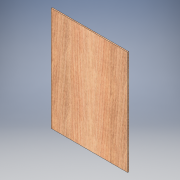
# Autodesk Inventor part: testBasePlate
Saved by Autodesk Inventor 2019 (Build 230136000, 136)
## iProperties
Created: 2019-02-01
Part Number: testBasePlate
Material: Wood (Birch)
Document SubType Name: Modeling
Designer: gaincarlo
Density: 0.55 g/cm^3
Appearance: Birch - Natural Polished
Author: gaincarlo
Autodesk Inventor part; units mm, degrees
ref_plane "YZ Plane" through (0, 0, 0) normal (1, 0, 0) x (0, 1, 0)
ref_plane "XZ Plane" through (0, 0, 0) normal (0, 1, 0) x (-1, 0, 0)
ref_plane "XY Plane" through (0, 0, 0) normal (0, 0, 1) x (1, 0, 0)
sketch "Sketch1" plane through (0, 0, 0) normal (0, 0, 1) x (1, 0, 0)
  line L0 (-165, 225) -> (165, 225)
  line L1 (165, 225) -> (165, -225)
  line L2 (165, -225) -> (-165, -225)
  line L3 (-165, -225) -> (-165, 225)
  line L4 (-231, 0) -> (231, 0) projected
  line L5 (0, -315) -> (0, 315) projected
  point P0 (0, 0)
  point P1 (-165, 0)
  point P2 (0, -225)
  dimension "d0" = 330
  dimension "d1" = 450
  constraints: 8 end point, 2 midpoint, 2 parallel, 2 point on line, 1 horizontal, 1 perpendicular
  measures "d0" distance of L1.end L2.end
  measures "d1" distance of L0.end L1.end
extrude "Extrusion1" add sketch "Sketch1" along normal blind 5
body "Solid1"
